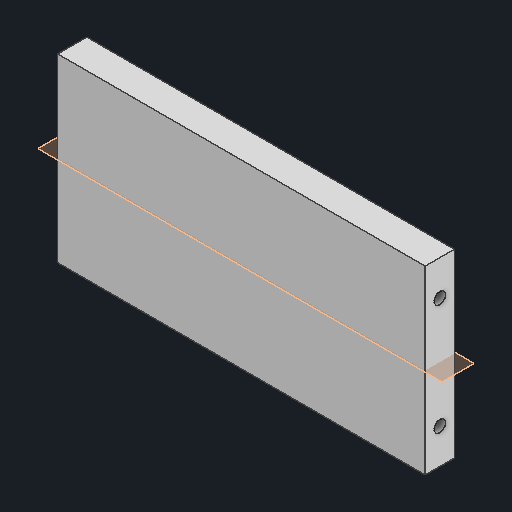
# Autodesk Inventor part: basetemplate
Saved by Autodesk Inventor 2026 (Build 300175000, 175)
## iProperties
Created: 2026-08-17
Part Number: basetemplate
Material: Generic
Document SubType Name: Modeling
Designer: imcle
Density: 1 g/cm^3
Appearance: Default
Author: imcle
Autodesk Inventor part; units mm, degrees
ref_plane "YZ Plane" through (0, 0, 0) normal (1, 0, 0) x (0, 1, 0)
ref_plane "XZ Plane" through (0, 0, 0) normal (0, 1, 0) x (-1, 0, 0)
ref_plane "XY Plane" through (0, 0, 0) normal (0, 0, 1) x (1, 0, 0)
sketch "Sketch1" plane through (0, 0, 0) normal (0, 0, 1) x (1, 0, 0)
  line L0 (-63, 30) -> (63, 30)
  line L1 (63, 30) -> (63, -30)
  line L2 (63, -30) -> (-63, -30)
  line L3 (-63, -30) -> (-63, 30)
  line L4 (-63, 30) -> (63, -30) construction
  line L5 (63, 30) -> (-63, -30) construction
  line L6 (-63, 30) -> (63, 30) construction
  point P0 (0, 0)
  dimension "d0" = 126
  dimension "d1" = 0
  dimension "d2" = 60
  constraints: 14 end point, 2 horizontal, 2 midpoint, 2 parallel, 1 collinear, 1 perpendicular
  measures "d0" distance of L0.start L0.end
  measures "d1" distance between parallel lines of L0 L6
  measures "d2" distance of L0.end L1.end
extrude "Extrusion1" add sketch "Sketch1" along normal blind 10
sketch "Sketch2" plane through (-63, -30, 0) normal (-1, 0, 0) x (0, 0, 1)
  line L0 (0, 60) -> (10, 60) projected
  line L1 (5, 60) -> (5, 49)
  circle A0 centre (5, 49) radius 2
  point P0 (0, 30)
  dimension "d5" = 11
  dimension "d6" = 4
  constraints: 2 end point, 1 centre point, 1 coincident, 1 midpoint, 1 vertical
  measures "d5" distance of L1.start L1.end
  measures "d6" diameter of A0
extrude "Extrusion2" cut sketch "Sketch2" against normal blind 5.5
pattern_linear "Rectangular Pattern1" count 2 spacing 120.5 along (1, 0, 0) count 2 spacing -38 along (0, 1, 0) of "Extrusion2"
ref_plane "Work Plane1" through (-63, 0, 0) normal (0, 1, 0) x (1, 0, 0)
sketch "Sketch3" plane through (-63, -30, 0) normal (0, -1, 0) x (1, 0, 0)
  line L0 (0, 0) -> (0, 10) projected
  line L1 (126, 0) -> (0, 0) projected
  line L2 (0, 10) -> (126, 10)
  line L3 (126, 10) -> (126, 0)
  line L4 (126, 0) -> (0, 0)
  line L5 (0, 0) -> (0, 10)
  point P0 (63, 0)
  constraints: 8 end point, 2 parallel, 1 horizontal, 1 perpendicular
extrude "Extrusion3" add sketch "Sketch3" along normal blind 1
mirror "Mirror1" about plane through (-63, 0, 0) normal (0, 1, 0) of "Extrusion3"
body "Solid1"
